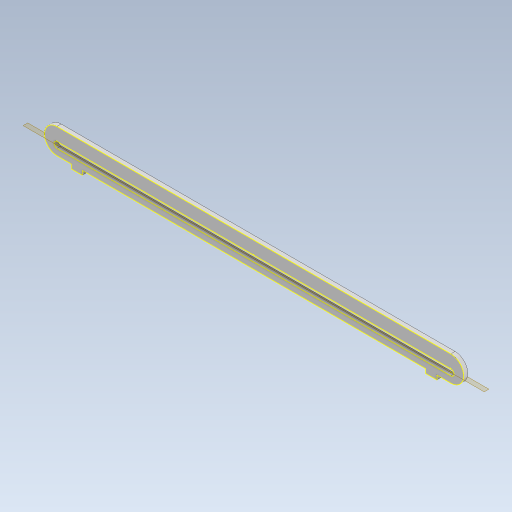
# Autodesk Inventor part: 零件4
Saved by Autodesk Inventor 2023 (Build 270158000, 158)
## iProperties
Created: 2023-04-16
Part Number: 零件4
Material: 一般
Document SubType Name: Modeling
Designer: JOU
Density: 1 g/cm^3
Appearance: 預設
Author: JOU
Autodesk Inventor part; units mm, degrees
ref_plane "YZ Plane" through (0, 0, 0) normal (1, 0, 0) x (0, 1, 0)
ref_plane "XZ Plane" through (0, 0, 0) normal (0, 1, 0) x (-1, 0, 0)
ref_plane "XY Plane" through (0, 0, 0) normal (0, 0, 1) x (1, 0, 0)
sketch "草圖1" plane through (0, 0, 0) normal (0, 0, 1) x (1, 0, 0)
  line L0 (-140, 0) -> (140, 0) construction
  line L1 (-140, 0) -> (140, 0) construction
  line L2 (-140, -9) -> (140, -9)
  line L3 (140, 9) -> (-140, 9)
  arc A0 (-140, 9) -> (-140, -9) centre (-140, 0) ccw
  arc A1 (140, -9) -> (140, 9) centre (140, 0) ccw
  line L4 (-140, -2.35) -> (140, -2.35) construction
  line L5 (-140, -4.5) -> (140, -4.5)
  line L6 (140, -0.2) -> (-140, -0.2)
  arc A2 (-140, -0.2) -> (-140, -4.5) centre (-140, -2.35) ccw
  arc A3 (140, -4.5) -> (140, -0.2) centre (140, -2.35) ccw
  line L7 (140, -2.35) -> (140, 0) construction
  point P0 (0, 0)
  point P1 (0, 0)
  point P2 (0, 0)
  point P3 (0, -2.35)
  dimension "d5" = 9
  dimension "d7" = 280
  dimension "d22" = 2.15
  dimension "d24" = 4.5
  constraints: 22 end point, 8 point on circle, 8 tangent, 4 centre point, 4 parallel, 3 midpoint, 2 coincident, 2 point on line, 1 horizontal, 1 vertical, 1 vertical alignment
  measures "d5" radius of A0
  measures "d7" distance of L1.end L1.start
  measures "d22" radius of A3
  measures "d24" distance between parallel lines of L2 L5
extrude "擠出1" add sketch "草圖1" along normal blind 3
sketch "草圖2" plane through (0, 0, 3) normal (0, 0, 1) x (1, 0, 0)
  line L0 (-208.6, 0) -> (208.6, 0) projected
  line L1 (-130, -9) -> (-122, -9)
  line L2 (-122, -9) -> (-122, -12)
  line L3 (-122, -12) -> (-130, -12)
  line L4 (-130, -12) -> (-130, -9)
  line L5 (122, -9) -> (130, -9)
  line L6 (130, -9) -> (130, -12)
  line L7 (130, -12) -> (122, -12)
  line L8 (122, -12) -> (122, -9)
  line L9 (-140, -9) -> (140, -9) projected
  point P0 (0, 0)
  dimension "d16" = 10
  dimension "d17" = 8
  dimension "d18" = 3
  dimension "d19" = 3
  dimension "d20" = 8
  dimension "d21" = 10
  constraints: 16 end point, 5 perpendicular, 2 collinear, 1 parallel
  measures "d16" distance from line of L4 L9.start
  measures "d17" distance of L2.end L3.end
  measures "d18" distance of L1.end L2.end
  measures "d19" distance of L5.end L6.end
  measures "d20" distance of L6.end L7.end
  measures "d21" distance from line of L9.end L6
extrude "擠出2" add sketch "草圖2" against normal up to surface (3 mm away)
ref_plane "工作平面2" through (-140, -2.35, 0) normal (0, 1, 0) x (1, 0, 0)
sketch "草圖3" plane through (0, 0, 3) normal (0, 0, 1) x (1, 0, 0)
  arc A0 (140, -9) -> (140, 9) centre (140, 0) ccw projected
  line L0 (140, 9) -> (-140, 9) projected
  arc A1 (-140, 9) -> (-140, -9) centre (-140, 0) ccw projected
  line L1 (-140, -9) -> (-130, -9) projected
  line L2 (-130, -9) -> (-130, -12) projected
  line L3 (-130, -12) -> (-122, -12) projected
  line L4 (-122, -12) -> (-122, -9) projected
  line L5 (-122, -9) -> (122, -9) projected
  line L6 (122, -9) -> (122, -12) projected
  line L7 (122, -12) -> (130, -12) projected
  line L8 (130, -12) -> (130, -9) projected
  line L9 (130, -9) -> (140, -9) projected
  arc A2 (-140, -0.2) -> (-140, -4.5) centre (-140, -2.35) ccw projected
  line L10 (-140, -0.2) -> (140, -0.2) projected
  arc A3 (140, -4.5) -> (140, -0.2) centre (140, -2.35) ccw projected
  line L11 (140, -4.5) -> (-140, -4.5) projected
  point P0 (0, 0)
